Autodesk Fusion 360 part; units mm, degrees
note: some values were not read from the file. Set by a fixed rule: which sketch regions a step uses.
(part 8 of 8)
  spline S993 degree 3 poles (32.1302, -141.7141) (30.6727, -141.6498) (29.2625, -140.8361) (28.4332, -139.581) knots 0 0 0 0 1 1 1 1
  spline S994 degree 3 poles (28.4332, -139.581) (28.0147, -138.9475) (27.7402, -138.2106) (27.6387, -137.4479) knots 0 0 0 0 1 1 1 1
  line L287 (27.6387, -137.4479) -> (27.2253, -124.3326)
  spline S995 degree 3 poles (27.2253, -124.3326) (27.261, -124.1184) (27.1963, -123.8884) (27.0555, -123.7285) knots 0 0 0 0 1 1 1 1
  spline S996 degree 3 poles (27.0555, -123.7285) (26.9778, -123.6402) (26.8783, -123.573) (26.7694, -123.5352) knots 0 0 0 0 1 1 1 1
  spline S997 degree 3 poles (26.7694, -123.5352) (26.6605, -123.4974) (26.5423, -123.489) (26.4295, -123.5111) knots 0 0 0 0 1 1 1 1
  line L288 (26.4295, -123.5111) -> (23.6519, -123.7321)
  spline S998 degree 3 poles (23.6519, -123.7321) (23.5393, -123.6984) (23.4178, -123.6981) (23.3051, -123.7312) knots 0 0 0 0 1 1 1 1
  spline S999 degree 3 poles (23.3051, -123.7312) (23.1924, -123.7643) (23.0888, -123.8306) (23.0094, -123.9206) knots 0 0 0 0 1 1 1 1
  spline S1000 degree 3 poles (23.0094, -123.9206) (22.8811, -124.0659) (22.8198, -124.273) (22.8472, -124.4687) knots 0 0 0 0 1 1 1 1
  line L289 (22.8472, -124.4687) -> (22.8987, -126.766)
  spline S1001 degree 3 poles (36.4911, -133.5813) (36.3024, -133.5736) (36.1111, -133.6504) (35.9788, -133.7913) knots 0 0 0 0 1 1 1 1
  spline S1002 degree 3 poles (35.9788, -133.7913) (35.8464, -133.9322) (35.776, -134.1353) (35.7946, -134.3318) knots 0 0 0 0 1 1 1 1
  spline S1003 degree 3 poles (35.7946, -134.3318) (35.8111, -134.5063) (35.8966, -134.672) (36.0252, -134.7844) knots 0 0 0 0 1 1 1 1
  spline S1004 degree 3 poles (36.0252, -134.7844) (36.1538, -134.8969) (36.3237, -134.9556) (36.4911, -134.9483) knots 0 0 0 0 1 1 1 1
  spline S1005 degree 3 poles (36.4911, -134.9483) (36.6536, -134.9417) (36.8134, -134.8725) (36.9315, -134.7557) knots 0 0 0 0 1 1 1 1
  spline S1006 degree 3 poles (36.9315, -134.7557) (37.0496, -134.6389) (37.1245, -134.4747) (37.1341, -134.305) knots 0 0 0 0 1 1 1 1
  spline S1007 degree 3 poles (37.1341, -134.305) (37.1446, -134.122) (37.0785, -133.9362) (36.9584, -133.8026) knots 0 0 0 0 1 1 1 1
  spline S1008 degree 3 poles (36.9584, -133.8026) (36.8383, -133.669) (36.6663, -133.5888) (36.4911, -133.5813) knots 0 0 0 0 1 1 1 1
  spline S1009 degree 3 poles (46.9493, -133.8297) (46.7703, -133.822) (46.5905, -133.904) (46.4712, -134.0437) knots 0 0 0 0 1 1 1 1
  spline S1010 degree 3 poles (46.4712, -134.0437) (46.3518, -134.1834) (46.294, -134.3772) (46.3113, -134.5636) knots 0 0 0 0 1 1 1 1
  spline S1011 degree 3 poles (46.3113, -134.5636) (46.3267, -134.7281) (46.3999, -134.8866) (46.5162, -134.9984) knots 0 0 0 0 1 1 1 1
  spline S1012 degree 3 poles (46.5162, -134.9984) (46.6326, -135.1102) (46.7914, -135.1734) (46.9493, -135.1665) knots 0 0 0 0 1 1 1 1
  spline S1013 degree 3 poles (46.9493, -135.1665) (47.1029, -135.1599) (47.2524, -135.0871) (47.3591, -134.9713) knots 0 0 0 0 1 1 1 1
  spline S1014 degree 3 poles (47.3591, -134.9713) (47.4657, -134.8554) (47.5292, -134.698) (47.5381, -134.5374) knots 0 0 0 0 1 1 1 1
  spline S1015 degree 3 poles (47.5381, -134.5374) (47.5477, -134.3637) (47.4929, -134.1862) (47.3847, -134.0539) knots 0 0 0 0 1 1 1 1
  spline S1016 degree 3 poles (47.3847, -134.0539) (47.2765, -133.9217) (47.1155, -133.8371) (46.9493, -133.8297) knots 0 0 0 0 1 1 1 1
  spline S1017 degree 3 poles (57.3652, -134.113) (57.1862, -134.1053) (57.0065, -134.1873) (56.8871, -134.327) knots 0 0 0 0 1 1 1 1
  spline S1018 degree 3 poles (56.8871, -134.327) (56.7678, -134.4668) (56.7099, -134.6605) (56.7273, -134.847) knots 0 0 0 0 1 1 1 1
  spline S1019 degree 3 poles (56.7273, -134.847) (56.7426, -135.0114) (56.8159, -135.1699) (56.9322, -135.2817) knots 0 0 0 0 1 1 1 1
  spline S1020 degree 3 poles (56.9322, -135.2817) (57.0485, -135.3935) (57.2073, -135.4567) (57.3652, -135.4498) knots 0 0 0 0 1 1 1 1
  spline S1021 degree 3 poles (57.3652, -135.4498) (57.5189, -135.4432) (57.6683, -135.3705) (57.775, -135.2546) knots 0 0 0 0 1 1 1 1
  spline S1022 degree 3 poles (57.775, -135.2546) (57.8817, -135.1387) (57.9452, -134.9813) (57.954, -134.8208) knots 0 0 0 0 1 1 1 1
  spline S1023 degree 3 poles (57.954, -134.8208) (57.9637, -134.647) (57.9088, -134.4695) (57.8006, -134.3372) knots 0 0 0 0 1 1 1 1
  spline S1024 degree 3 poles (57.8006, -134.3372) (57.6925, -134.205) (57.5315, -134.1204) (57.3652, -134.113) knots 0 0 0 0 1 1 1 1
  spline S1025 degree 3 poles (101.665, -134.9463) (101.4861, -134.9385) (101.3063, -135.0206) (101.187, -135.1603) knots 0 0 0 0 1 1 1 1
  spline S1026 degree 3 poles (101.187, -135.1603) (101.0676, -135.3) (101.0097, -135.4938) (101.0271, -135.6802) knots 0 0 0 0 1 1 1 1
  spline S1027 degree 3 poles (101.0271, -135.6802) (101.0425, -135.8446) (101.1157, -136.0032) (101.232, -136.115) knots 0 0 0 0 1 1 1 1
  spline S1028 degree 3 poles (101.232, -136.115) (101.3483, -136.2268) (101.5072, -136.2899) (101.665, -136.2831) knots 0 0 0 0 1 1 1 1
  spline S1029 degree 3 poles (101.665, -136.2831) (101.8187, -136.2765) (101.9682, -136.2037) (102.0748, -136.0879) knots 0 0 0 0 1 1 1 1
  spline S1030 degree 3 poles (102.0748, -136.0879) (102.1815, -135.972) (102.245, -135.8146) (102.2539, -135.654) knots 0 0 0 0 1 1 1 1
  spline S1031 degree 3 poles (102.2539, -135.654) (102.2635, -135.4803) (102.2086, -135.3027) (102.1005, -135.1705) knots 0 0 0 0 1 1 1 1
  spline S1032 degree 3 poles (102.1005, -135.1705) (101.9923, -135.0382) (101.8313, -134.9537) (101.665, -134.9463) knots 0 0 0 0 1 1 1 1
  spline S1033 degree 3 poles (111.9273, -135.1463) (111.7483, -135.1385) (111.5686, -135.2206) (111.4492, -135.3603) knots 0 0 0 0 1 1 1 1
  spline S1034 degree 3 poles (111.4492, -135.3603) (111.3299, -135.5) (111.272, -135.6938) (111.2894, -135.8802) knots 0 0 0 0 1 1 1 1
  spline S1035 degree 3 poles (111.2894, -135.8802) (111.3047, -136.0446) (111.378, -136.2032) (111.4943, -136.315) knots 0 0 0 0 1 1 1 1
  spline S1036 degree 3 poles (111.4943, -136.315) (111.6106, -136.4268) (111.7695, -136.4899) (111.9273, -136.4831) knots 0 0 0 0 1 1 1 1
  spline S1037 degree 3 poles (111.9273, -136.4831) (112.081, -136.4764) (112.2304, -136.4037) (112.3371, -136.2878) knots 0 0 0 0 1 1 1 1
  spline S1038 degree 3 poles (112.3371, -136.2878) (112.4438, -136.172) (112.5073, -136.0146) (112.5161, -135.854) knots 0 0 0 0 1 1 1 1
  spline S1039 degree 3 poles (112.5161, -135.854) (112.5257, -135.6802) (112.4709, -135.5027) (112.3627, -135.3705) knots 0 0 0 0 1 1 1 1
  spline S1040 degree 3 poles (112.3627, -135.3705) (112.2546, -135.2382) (112.0936, -135.1537) (111.9273, -135.1463) knots 0 0 0 0 1 1 1 1
  spline S1041 degree 2 poles (10.837, -247.6762) (10.81, -245.3593) (10.8501, -244.0773) knots 0 0 0 1 1 1
  spline S1042 degree 3 poles (10.8501, -244.0773) (10.8548, -243.9237) (11.0104, -243.7661) (11.2499, -243.7651) knots 0 0 0 0 1 1 1 1
  spline S1043 degree 3 poles (11.2499, -243.7651) (11.7315, -243.7632) (12.7052, -243.7841) (13.0357, -243.7851) knots 0 0 0 0 1 1 1 1
  spline S1044 degree 3 poles (13.0357, -243.7851) (13.2758, -243.786) (13.4047, -243.6398) (13.4067, -243.5043) knots 0 0 0 0 1 1 1 1
  spline S1045 degree 3 poles (13.4067, -243.5043) (13.4381, -241.3814) (13.4313, -241.3803) (13.4631, -238.9109) knots 0 0 0 0 1 1 1 1
  spline S1046 degree 3 poles (13.4631, -238.9109) (13.4659, -238.6921) (13.2899, -238.5225) (13.0138, -238.5197) knots 0 0 0 0 1 1 1 1
  spline S1047 degree 3 poles (13.0138, -238.5197) (11.7178, -238.5066) (11.93, -238.5149) (11.2628, -238.512) knots 0 0 0 0 1 1 1 1
  spline S1048 degree 3 poles (11.2628, -238.512) (11.1347, -238.5115) (11.0448, -238.4159) (11.0435, -238.2054) knots 0 0 0 0 1 1 1 1
  spline S1049 degree 3 poles (11.0435, -238.2054) (11.0341, -236.7209) (11.0102, -236.7243) (11.0082, -234.862) knots 0 0 0 0 1 1 1 1
  spline S1050 degree 3 poles (11.0082, -234.862) (11.008, -234.6358) (10.9701, -234.5433) (11.2164, -234.546) knots 0 0 0 0 1 1 1 1
  line L290 (11.2164, -234.546) -> (17.2284, -234.6114)
  spline S1051 degree 3 poles (17.2284, -234.6114) (17.5142, -234.6143) (17.5959, -234.6922) (17.5893, -234.9527) knots 0 0 0 0 1 1 1 1
  spline S1052 degree 3 poles (17.5893, -234.9527) (17.5714, -235.6578) (17.819, -236.1257) (18.8656, -236.1706) knots 0 0 0 0 1 1 1 1
  line L291 (18.8656, -236.1706) -> (20.0607, -236.1764)
  spline S1053 degree 2 poles (20.0607, -236.1764) (20.0909, -238.4972) (20.1073, -239.6995) knots 0 0 0 1 1 1
  spline S1054 degree 3 poles (20.1073, -239.6995) (20.109, -239.824) (19.923, -239.9537) (19.7659, -239.9573) knots 0 0 0 0 1 1 1 1
  spline S1055 degree 3 poles (19.7659, -239.9573) (19.0783, -239.9729) (19.0691, -239.9919) (18.4394, -239.9861) knots 0 0 0 0 1 1 1 1
  spline S1056 degree 3 poles (18.4394, -239.9861) (18.2321, -239.9842) (17.9896, -240.1446) (17.9938, -240.3088) knots 0 0 0 0 1 1 1 1
  spline S1057 degree 3 poles (17.9938, -240.3088) (18.0237, -241.5017) (18.0241, -241.5062) (18.0726, -243.1232) knots 0 0 0 0 1 1 1 1
  spline S1058 degree 3 poles (18.0726, -243.1232) (18.0757, -243.2251) (17.962, -243.3631) (17.8333, -243.3632) knots 0 0 0 0 1 1 1 1
  spline S1059 degree 3 poles (17.8333, -243.3632) (17.5642, -243.3634) (17.4937, -243.37) (17.2055, -243.3763) knots 0 0 0 0 1 1 1 1
  spline S1060 degree 3 poles (17.2055, -243.3763) (17.0597, -243.3792) (16.9227, -243.5059) (16.9245, -243.6146) knots 0 0 0 0 1 1 1 1
  line L292 (16.9245, -243.6146) -> (16.9899, -247.6918)
  line L293 (16.9899, -247.6918) -> (10.837, -247.6762)
  spline S1061 degree 2 poles (47.8882, -247.7867) (47.859, -245.8925) (47.8189, -244.6105) knots 0 0 0 1 1 1
  spline S1062 degree 3 poles (47.8189, -244.6105) (47.8142, -244.4569) (47.6586, -244.2992) (47.4191, -244.2983) knots 0 0 0 0 1 1 1 1
  spline S1063 degree 3 poles (47.4191, -244.2983) (46.9375, -244.2963) (45.9638, -244.3173) (45.6333, -244.3182) knots 0 0 0 0 1 1 1 1
  spline S1064 degree 3 poles (45.6333, -244.3182) (45.3932, -244.3192) (45.2643, -244.173) (45.2623, -244.0375) knots 0 0 0 0 1 1 1 1
  spline S1065 degree 3 poles (45.2623, -244.0375) (45.2309, -241.9146) (45.2377, -241.9135) (45.2059, -239.444) knots 0 0 0 0 1 1 1 1
  spline S1066 degree 3 poles (45.2059, -239.444) (45.2031, -239.2253) (45.3791, -239.0557) (45.6552, -239.0529) knots 0 0 0 0 1 1 1 1
  spline S1067 degree 3 poles (45.6552, -239.0529) (46.9512, -239.0398) (46.739, -239.0481) (47.4062, -239.0452) knots 0 0 0 0 1 1 1 1
  spline S1068 degree 3 poles (47.4062, -239.0452) (47.5343, -239.0447) (47.6242, -238.9491) (47.6255, -238.7386) knots 0 0 0 0 1 1 1 1
  spline S1069 degree 3 poles (47.6255, -238.7386) (47.6349, -237.254) (47.6588, -237.2575) (47.6608, -235.3952) knots 0 0 0 0 1 1 1 1
  spline S1070 degree 3 poles (47.6608, -235.3952) (47.661, -235.1689) (47.6989, -235.0765) (47.4526, -235.0791) knots 0 0 0 0 1 1 1 1
  line L294 (47.4526, -235.0791) -> (41.4406, -235.1446)
  spline S1071 degree 3 poles (41.4406, -235.1446) (41.1548, -235.1475) (41.1393, -235.1728) (41.1459, -235.4334) knots 0 0 0 0 1 1 1 1
  spline S1072 degree 3 poles (41.1459, -235.4334) (41.1638, -236.1385) (40.9162, -236.5277) (39.8696, -236.5726) knots 0 0 0 0 1 1 1 1
  line L295 (39.8696, -236.5726) -> (38.5255, -236.5259)
  spline S1073 degree 2 poles (38.5255, -236.5259) (38.5118, -238.5714) (38.4955, -239.7736) knots 0 0 0 1 1 1
  spline S1074 degree 3 poles (38.4955, -239.7736) (38.4938, -239.8982) (38.6797, -240.0279) (38.8369, -240.0315) knots 0 0 0 0 1 1 1 1
  spline S1075 degree 3 poles (38.8369, -240.0315) (39.5245, -240.0471) (39.0039, -240.053) (39.6336, -240.0472) knots 0 0 0 0 1 1 1 1
  spline S1076 degree 3 poles (39.6336, -240.0472) (39.8409, -240.0452) (40.0781, -240.2056) (40.0793, -240.3698) knots 0 0 0 0 1 1 1 1
  spline S1077 degree 3 poles (40.0793, -240.3698) (40.0997, -243.2891) (40.0793, -240.3698) (40.0997, -243.2891) knots 0 0 0 0 1 1 1 1
  spline S1078 degree 3 poles (40.0997, -243.2891) (40.1004, -243.3911) (40.2104, -243.5291) (40.3391, -243.5292) knots 0 0 0 0 1 1 1 1
  spline S1079 degree 3 poles (40.3391, -243.5292) (40.6082, -243.5294) (40.6787, -243.5359) (40.9668, -243.5422) knots 0 0 0 0 1 1 1 1
  spline S1080 degree 3 poles (40.9668, -243.5422) (41.1127, -243.5451) (41.2482, -243.6718) (41.2479, -243.7806) knots 0 0 0 0 1 1 1 1
  line L296 (41.2479, -243.7806) -> (41.2883, -247.7892)
  line L297 (41.2883, -247.7892) -> (47.8882, -247.7867)
  spline S1081 degree 3 poles (7.9694, -248.7095) (6.13, -246.5222) (6.2347, -236.0812) (8.0811, -233.6481) knots 0 0 0 0 1 1 1 1
  spline S1082 degree 3 poles (8.0811, -233.6481) (10.5104, -230.4468) (17.2788, -229.16) (22.0462, -228.4083) knots 0 0 0 0 1 1 1 1
  spline S1083 degree 3 poles (22.0462, -228.4083) (24.6723, -227.9942) (34.366, -228.0312) (36.3491, -228.4083) knots 0 0 0 0 1 1 1 1
  spline S1084 degree 3 poles (36.3491, -228.4083) (41.2162, -229.3338) (47.3408, -230.9515) (49.7581, -232.9453) knots 0 0 0 0 1 1 1 1
  spline S1085 degree 3 poles (49.7581, -232.9453) (52.8167, -235.4681) (52.4282, -246.7854) (50.3256, -249.234) knots 0 0 0 0 1 1 1 1
  spline S1086 degree 3 poles (50.3256, -249.234) (47.576, -252.4361) (40.6483, -252.9931) (35.4495, -254.2169) knots 0 0 0 0 1 1 1 1
  spline S1087 degree 3 poles (35.4495, -254.2169) (33.2181, -254.7421) (24.4667, -254.5045) (22.8569, -254.2015) knots 0 0 0 0 1 1 1 1
  spline S1088 degree 3 poles (22.8569, -254.2015) (17.5924, -253.2105) (10.1045, -251.2484) (7.9694, -248.7095) knots 0 0 0 0 1 1 1 1
  spline S1089 degree 3 poles (29.1976, -234.073) (31.1453, -234.0759) (32.8241, -235.8872) (32.8396, -237.6921) knots 0 0 0 0 1 1 1 1
  spline S1090 degree 3 poles (32.8396, -237.6921) (32.8528, -239.2378) (31.2151, -241.3793) (29.2639, -241.3637) knots 0 0 0 0 1 1 1 1
  spline S1091 degree 3 poles (29.2639, -241.3637) (27.2598, -241.3477) (25.6544, -239.1221) (25.6881, -237.5348) knots 0 0 0 0 1 1 1 1
  spline S1092 degree 3 poles (25.6881, -237.5348) (25.7252, -235.7929) (27.3293, -234.0703) (29.1976, -234.073) knots 0 0 0 0 1 1 1 1
  spline S1093 degree 3 poles (29.1645, -230.3227) (28.7036, -230.3295) (28.2258, -230.7707) (28.2375, -231.1357) knots 0 0 0 0 1 1 1 1
  spline S1094 degree 3 poles (28.2375, -231.1357) (28.2502, -231.5312) (28.7982, -231.9953) (29.297, -231.9749) knots 0 0 0 0 1 1 1 1
  spline S1095 degree 3 poles (29.297, -231.9749) (29.7514, -231.9564) (30.1775, -231.4958) (30.1578, -231.1357) knots 0 0 0 0 1 1 1 1
  spline S1096 degree 3 poles (30.1578, -231.1357) (30.1372, -230.759) (29.6406, -230.3162) (29.1645, -230.3227) knots 0 0 0 0 1 1 1 1
  spline S1097 degree 3 poles (29.0652, -243.4355) (28.6043, -243.4423) (28.1265, -243.8835) (28.1382, -244.2485) knots 0 0 0 0 1 1 1 1
  spline S1098 degree 3 poles (28.1382, -244.2485) (28.1509, -244.644) (28.6989, -245.1081) (29.1977, -245.0877) knots 0 0 0 0 1 1 1 1
  spline S1099 degree 3 poles (29.1977, -245.0877) (29.6521, -245.0692) (30.0782, -244.6086) (30.0585, -244.2485) knots 0 0 0 0 1 1 1 1
  spline S1100 degree 3 poles (30.0585, -244.2485) (30.0378, -243.8718) (29.5412, -243.429) (29.0652, -243.4355) knots 0 0 0 0 1 1 1 1
  spline S1101 degree 3 poles (22.5759, -236.748) (22.115, -236.7548) (21.6372, -237.1959) (21.6489, -237.561) knots 0 0 0 0 1 1 1 1
  spline S1102 degree 3 poles (21.6489, -237.561) (21.6616, -237.9565) (22.2096, -238.4206) (22.7084, -238.4002) knots 0 0 0 0 1 1 1 1
  spline S1103 degree 3 poles (22.7084, -238.4002) (23.1628, -238.3817) (23.5889, -237.9211) (23.5692, -237.561) knots 0 0 0 0 1 1 1 1
  spline S1104 degree 3 poles (23.5692, -237.561) (23.5486, -237.1842) (23.052, -236.7415) (22.5759, -236.748) knots 0 0 0 0 1 1 1 1
  spline S1105 degree 3 poles (35.5545, -236.8267) (35.0935, -236.8334) (34.6157, -237.2746) (34.6275, -237.6397) knots 0 0 0 0 1 1 1 1
  spline S1106 degree 3 poles (34.6275, -237.6397) (34.6401, -238.0352) (35.1881, -238.4993) (35.6869, -238.4789) knots 0 0 0 0 1 1 1 1
  spline S1107 degree 3 poles (35.6869, -238.4789) (36.1414, -238.4604) (36.5675, -237.9998) (36.5477, -237.6397) knots 0 0 0 0 1 1 1 1
  spline S1108 degree 3 poles (36.5477, -237.6397) (36.5271, -237.2629) (36.0305, -236.8202) (35.5545, -236.8267) knots 0 0 0 0 1 1 1 1
  spline S1109 degree 3 poles (18.785, -250.3459) (18.748, -249.1063) (18.7991, -248.5212) (18.7685, -247.3694) knots 0 0 0 0 1 1 1 1
  spline S1110 degree 3 poles (18.7685, -247.3694) (18.7615, -247.1095) (18.9371, -246.8518) (19.381, -246.858) knots 0 0 0 0 1 1 1 1
  spline S1111 degree 3 poles (19.381, -246.858) (25.3461, -246.9402) (29.4591, -246.8339) (38.9481, -246.8579) knots 0 0 0 0 1 1 1 1
  spline S1112 degree 3 poles (38.9481, -246.8579) (39.4808, -246.8589) (39.8824, -246.9253) (39.8917, -247.2382) knots 0 0 0 0 1 1 1 1
  spline S1113 degree 3 poles (39.8917, -247.2382) (39.9326, -248.6175) (39.9249, -249.0855) (39.9579, -250.8311) knots 0 0 0 0 1 1 1 1
  spline S1114 degree 3 poles (39.9579, -250.8311) (39.9639, -251.1444) (39.3598, -251.1674) (38.8847, -251.1733) knots 0 0 0 0 1 1 1 1
  spline S1115 degree 3 poles (38.8847, -251.1733) (31.2086, -251.2686) (22.9608, -251.1294) (19.6127, -251.1458) knots 0 0 0 0 1 1 1 1
  spline S1116 degree 3 poles (19.6127, -251.1458) (18.9796, -251.1794) (18.7993, -250.8065) (18.785, -250.3459) knots 0 0 0 0 1 1 1 1
  spline S1117 degree 3 poles (106.8581, -62.4361) (107.4615, -63.4086) (126.8754, -59.2722) (130.1181, -59.5077) knots 0 0 0 0 1 1 1 1
  spline S1118 degree 3 poles (130.1181, -59.5077) (134.3606, -59.8157) (139.0785, -60.7934) (144.166, -60.6989) knots 0 0 0 0 1 1 1 1
  spline S1119 degree 3 poles (144.166, -60.6989) (145.4225, -60.6737) (146.6093, -58.2172) (146.1712, -58.2172) knots 0 0 0 0 1 1 1 1
  line L298 (146.1712, -58.2172) -> (144.4491, -58.1794)
  line L299 (144.4491, -58.1794) -> (144.5317, -54.8538)
  line L300 (144.5317, -54.8538) -> (148.9077, -54.8665)
  spline S1120 degree 3 poles (148.9077, -54.8665) (150.9289, -54.8707) (153.9314, -45.6994) (153.2011, -43.1776) knots 0 0 0 0 1 1 1 1
  spline S1121 degree 2 poles (153.2011, -43.1776) (152.9643, -42.3602) (131.8833, -41.4876) knots 0 0 0 1 1 1
  line L301 (131.8833, -41.4876) -> (132.3596, -27.2637)
  spline S1122 degree 2 poles (132.3596, -27.2637) (152.4979, -28.1981) (153.5195, -27.5927) knots 0 0 0 1 1 1
  spline S1123 degree 3 poles (153.5195, -27.5927) (155.6549, -26.3272) (151.6676, -14.9886) (150.4764, -14.9732) knots 0 0 0 0 1 1 1 1
  line L302 (150.4764, -14.9732) -> (146.6548, -14.9236)
  line L303 (146.6548, -14.9236) -> (146.6428, -11.4244)
  line L304 (146.6428, -11.4244) -> (147.9756, -11.4117)
  spline S1124 degree 2 poles (147.9756, -11.4117) (149.5302, -11.3991) (145.4515, -8.5825) knots 0 0 0 1 1 1
  spline S1125 degree 2 poles (145.4515, -8.5825) (137.5261, -9.626) (133.562, -9.3767) knots 0 0 0 1 1 1
  spline S1126 degree 3 poles (133.562, -9.3767) (125.1006, -8.8445) (109.1577, -3.6312) (108.5564, -4.5126) knots 0 0 0 0 1 1 1 1
  spline S1127 degree 3 poles (108.5564, -4.5126) (107.7409, -5.708) (114.1986, -16.9111) (115.5391, -23.5721) knots 0 0 0 0 1 1 1 1
  spline S1128 degree 2 poles (115.5391, -23.5721) (116.1079, -26.3984) (115.9459, -32.2282) knots 0 0 0 1 1 1
  line L305 (115.9459, -32.2282) -> (117.8444, -32.2313)
  line L306 (117.8444, -32.2313) -> (117.8981, -35.9809)
  line L307 (117.8981, -35.9809) -> (116.0412, -36.0359)
  spline S1129 degree 2 poles (116.0412, -36.0359) (116.1197, -41.6582) (115.256, -44.2203) knots 0 0 0 1 1 1
  spline S1130 degree 3 poles (115.256, -44.2203) (113.7246, -48.7631) (106.2438, -61.4466) (106.8581, -62.4361) knots 0 0 0 0 1 1 1 1
  spline S1131 degree 3 poles (118.1745, -48.0159) (119.0012, -48.0327) (125.7923, -54.9365) (125.5975, -56.246) knots 0 0 0 0 1 1 1 1
  spline S1132 degree 3 poles (125.5975, -56.246) (125.4017, -57.5625) (113.7841, -58.9903) (113.0869, -57.9833) knots 0 0 0 0 1 1 1 1
  spline S1133 degree 3 poles (113.0869, -57.9833) (112.4893, -57.1201) (117.1764, -47.9978) (118.1745, -48.0159) knots 0 0 0 0 1 1 1 1
  spline S1134 degree 3 poles (115.2217, -9.406) (114.805, -10.0096) (118.3286, -19.4875) (119.2901, -19.5024) knots 0 0 0 0 1 1 1 1
  spline S1135 degree 3 poles (119.2901, -19.5024) (120.1689, -19.515) (127.7392, -13.1963) (127.3344, -11.8338) knots 0 0 0 0 1 1 1 1
  spline S1136 degree 3 poles (127.3344, -11.8338) (127.0183, -10.7697) (115.6902, -8.7274) (115.2217, -9.406) knots 0 0 0 0 1 1 1 1
  spline S1137 degree 3 poles (23.635, -150.8434) (24.5086, -148.6901) (26.1171, -146.8428) (28.1299, -145.6814) knots 0 0 0 0 1 1 1 1
  spline S1138 degree 3 poles (28.1299, -145.6814) (30.1426, -144.5201) (32.5469, -144.0519) (34.8484, -144.3733) knots 0 0 0 0 1 1 1 1
  spline S1139 degree 3 poles (34.8484, -144.3733) (52.6997, -145.8548) (70.5006, -147.9437) (88.21, -150.6351) knots 0 0 0 0 1 1 1 1
  spline S1140 degree 3 poles (88.21, -150.6351) (96.7525, -151.9334) (105.2738, -153.3718) (113.7692, -154.9496) knots 0 0 0 0 1 1 1 1
  line L308 (113.7692, -154.9496) -> (119.5937, -159.5032)
  spline S1141 degree 3 poles (119.5937, -159.5032) (120.3382, -160.7189) (120.741, -162.1415) (120.7442, -163.5672) knots 0 0 0 0 1 1 1 1
  spline S1142 degree 3 poles (120.7442, -163.5672) (120.7472, -164.9195) (120.3916, -166.2711) (119.7232, -167.4468) knots 0 0 0 0 1 1 1 1
  line L309 (119.7232, -167.4468) -> (112.4351, -171.7089)
  spline S1143 degree 3 poles (112.4351, -171.7089) (103.5371, -171.4668) (94.6435, -171.0669) (85.7597, -170.5096) knots 0 0 0 0 1 1 1 1
  spline S1144 degree 3 poles (85.7597, -170.5096) (67.4605, -169.3616) (49.2034, -167.5449) (31.0368, -165.0646) knots 0 0 0 0 1 1 1 1
  spline S1145 degree 3 poles (31.0368, -165.0646) (28.0767, -164.3852) (25.4542, -162.3573) (24.052, -159.6632) knots 0 0 0 0 1 1 1 1
  spline S1146 degree 3 poles (24.052, -159.6632) (22.6499, -156.9692) (22.4933, -153.6578) (23.635, -150.8434) knots 0 0 0 0 1 1 1 1
  spline S1147 degree 3 poles (26.953, -153.0854) (26.6067, -153.0691) (26.2584, -153.2223) (26.0288, -153.4822) knots 0 0 0 0 1 1 1 1
  spline S1148 degree 3 poles (26.0288, -153.4822) (25.7992, -153.7422) (25.6904, -154.102) (25.7279, -154.4467) knots 0 0 0 0 1 1 1 1
  spline S1149 degree 3 poles (25.7279, -154.4467) (25.7605, -154.7462) (25.9022, -155.0338) (26.1254, -155.236) knots 0 0 0 0 1 1 1 1
  spline S1150 degree 3 poles (26.1254, -155.236) (26.3486, -155.4381) (26.6523, -155.5509) (26.953, -155.5358) knots 0 0 0 0 1 1 1 1
  spline S1151 degree 3 poles (26.953, -155.5358) (27.2117, -155.5236) (27.4635, -155.4156) (27.657, -155.2433) knots 0 0 0 0 1 1 1 1
  spline S1152 degree 3 poles (27.657, -155.2433) (27.8504, -155.0709) (27.9852, -154.8355) (28.042, -154.5828) knots 0 0 0 0 1 1 1 1
  spline S1153 degree 3 poles (28.042, -154.5828) (28.1192, -154.2398) (28.049, -153.8643) (27.8451, -153.578) knots 0 0 0 0 1 1 1 1
  spline S1154 degree 3 poles (27.8451, -153.578) (27.6411, -153.2916) (27.3042, -153.1017) (26.953, -153.0854) knots 0 0 0 0 1 1 1 1
  spline S1155 degree 3 poles (48.9034, -160.1299) (48.8627, -160.2823) (48.8293, -160.4376) (48.8273, -160.5953) knots 0 0 0 0 1 1 1 1
  spline S1156 degree 3 poles (48.8273, -160.5953) (48.8253, -160.753) (48.8562, -160.9135) (48.9377, -161.0488) knots 0 0 0 0 1 1 1 1
  spline S1157 degree 3 poles (48.9377, -161.0488) (49.0524, -161.2395) (49.2679, -161.3654) (49.4903, -161.3719) knots 0 0 0 0 1 1 1 1
  spline S1158 degree 3 poles (49.4903, -161.3719) (49.7127, -161.38) (49.9351, -161.2651) (50.0607, -161.0814) knots 0 0 0 0 1 1 1 1
  spline S1159 degree 3 poles (50.0607, -161.0814) (51.4229, -159.8943) (52.2579, -158.123) (52.3068, -156.3169) knots 0 0 0 0 1 1 1 1
  spline S1160 degree 3 poles (52.3068, -156.3169) (52.3439, -154.9506) (51.9504, -153.5989) (51.3539, -152.3692) knots 0 0 0 0 1 1 1 1
  spline S1161 degree 3 poles (51.3539, -152.3692) (51.2759, -152.2082) (51.1934, -152.0477) (51.0788, -151.9107) knots 0 0 0 0 1 1 1 1
  spline S1162 degree 3 poles (51.0788, -151.9107) (50.9641, -151.7738) (50.8134, -151.6606) (50.6393, -151.6206) knots 0 0 0 0 1 1 1 1
  spline S1163 degree 3 poles (50.6393, -151.6206) (50.5334, -151.5962) (50.4213, -151.6003) (50.3173, -151.6329) knots 0 0 0 0 1 1 1 1
  spline S1164 degree 3 poles (50.3173, -151.6329) (50.2133, -151.6655) (50.1177, -151.7225) (50.0426, -151.8012) knots 0 0 0 0 1 1 1 1
  spline S1165 degree 3 poles (50.0426, -151.8012) (49.9676, -151.8798) (49.9133, -151.978) (49.8868, -152.0832) knots 0 0 0 0 1 1 1 1
  spline S1166 degree 3 poles (49.8868, -152.0832) (49.8603, -152.1883) (49.8615, -152.3008) (49.8906, -152.405) knots 0 0 0 0 1 1 1 1
  spline S1167 degree 3 poles (49.8906, -152.405) (50.1218, -153.7984) (50.1335, -155.228) (49.9248, -156.625) knots 0 0 0 0 1 1 1 1
  spline S1168 degree 3 poles (49.9248, -156.625) (49.7444, -157.8322) (49.4, -159.015) (48.9038, -160.1302) knots 0 0 0 0 1 1 1 1
  spline S1169 degree 3 poles (48.9038, -160.1302) (48.9037, -160.1307) (48.9036, -160.1312) (48.9035, -160.1317) knots 0 0 0 0 1 1 1 1
  line L310 (48.9035, -160.1317) -> (48.9034, -160.1299)
  spline S1170 degree 3 poles (61.3829, -161.6031) (61.3422, -161.7554) (61.3088, -161.9107) (61.3068, -162.0684) knots 0 0 0 0 1 1 1 1
  spline S1171 degree 3 poles (61.3068, -162.0684) (61.3047, -162.2261) (61.3357, -162.3866) (61.4171, -162.5219) knots 0 0 0 0 1 1 1 1
  spline S1172 degree 3 poles (61.4171, -162.5219) (61.5319, -162.7126) (61.7473, -162.8385) (61.9698, -162.845) knots 0 0 0 0 1 1 1 1
  spline S1173 degree 3 poles (61.9698, -162.845) (62.1922, -162.8532) (62.4146, -162.7383) (62.5402, -162.5545) knots 0 0 0 0 1 1 1 1
  spline S1174 degree 3 poles (62.5402, -162.5545) (63.9023, -161.3674) (64.7374, -159.5962) (64.7863, -157.79) knots 0 0 0 0 1 1 1 1
  spline S1175 degree 3 poles (64.7863, -157.79) (64.8233, -156.4237) (64.4299, -155.0721) (63.8334, -153.8423) knots 0 0 0 0 1 1 1 1
  spline S1176 degree 3 poles (63.8334, -153.8423) (63.7554, -153.6814) (63.6729, -153.5208) (63.5582, -153.3839) knots 0 0 0 0 1 1 1 1
  spline S1177 degree 3 poles (63.5582, -153.3839) (63.4436, -153.247) (63.2929, -153.1337) (63.1187, -153.0938) knots 0 0 0 0 1 1 1 1
  spline S1178 degree 3 poles (63.1187, -153.0938) (63.0129, -153.0693) (62.9008, -153.0734) (62.7968, -153.106) knots 0 0 0 0 1 1 1 1
  spline S1179 degree 3 poles (62.7968, -153.106) (62.6928, -153.1386) (62.5971, -153.1957) (62.5221, -153.2743) knots 0 0 0 0 1 1 1 1
  spline S1180 degree 3 poles (62.5221, -153.2743) (62.447, -153.353) (62.3928, -153.4512) (62.3663, -153.5563) knots 0 0 0 0 1 1 1 1
  spline S1181 degree 3 poles (62.3663, -153.5563) (62.3398, -153.6614) (62.341, -153.7739) (62.37, -153.8782) knots 0 0 0 0 1 1 1 1
  spline S1182 degree 3 poles (62.37, -153.8782) (62.6013, -155.2715) (62.6129, -156.7011) (62.4043, -158.0981) knots 0 0 0 0 1 1 1 1
  spline S1183 degree 3 poles (62.4043, -158.0981) (62.2239, -159.3054) (61.8795, -160.4881) (61.3833, -161.6034) knots 0 0 0 0 1 1 1 1
  spline S1184 degree 3 poles (61.3833, -161.6034) (61.3832, -161.6039) (61.383, -161.6044) (61.3829, -161.6049) knots 0 0 0 0 1 1 1 1
  line L311 (61.3829, -161.6049) -> (61.3829, -161.6031)
  spline S1185 degree 3 poles (73.8962, -162.8544) (73.8554, -163.0067) (73.822, -163.162) (73.82, -163.3197) knots 0 0 0 0 1 1 1 1
  spline S1186 degree 3 poles (73.82, -163.3197) (73.818, -163.4774) (73.849, -163.6384) (73.9304, -163.7732) knots 0 0 0 0 1 1 1 1
  spline S1187 degree 3 poles (73.9304, -163.7732) (74.0452, -163.9639) (74.2606, -164.0898) (74.483, -164.0963) knots 0 0 0 0 1 1 1 1
  spline S1188 degree 3 poles (74.483, -164.0963) (74.7055, -164.1045) (74.9278, -163.9896) (75.0535, -163.8058) knots 0 0 0 0 1 1 1 1
  spline S1189 degree 3 poles (75.0535, -163.8058) (76.4156, -162.6187) (77.2506, -160.8475) (77.2995, -159.0413) knots 0 0 0 0 1 1 1 1
  spline S1190 degree 3 poles (77.2995, -159.0413) (77.3366, -157.675) (76.9432, -156.3234) (76.3467, -155.0936) knots 0 0 0 0 1 1 1 1
  spline S1191 degree 3 poles (76.3467, -155.0936) (76.2687, -154.9327) (76.1862, -154.7721) (76.0715, -154.6352) knots 0 0 0 0 1 1 1 1
  spline S1192 degree 3 poles (76.0715, -154.6352) (75.9568, -154.4983) (75.8062, -154.385) (75.632, -154.3451) knots 0 0 0 0 1 1 1 1
  spline S1193 degree 3 poles (75.632, -154.3451) (75.5262, -154.3206) (75.414, -154.3247) (75.3101, -154.3573) knots 0 0 0 0 1 1 1 1
  spline S1194 degree 3 poles (75.3101, -154.3573) (75.206, -154.3899) (75.1104, -154.447) (75.0354, -154.5256) knots 0 0 0 0 1 1 1 1
  spline S1195 degree 3 poles (75.0354, -154.5256) (74.9603, -154.6043) (74.9061, -154.7024) (74.8795, -154.8076) knots 0 0 0 0 1 1 1 1
  spline S1196 degree 3 poles (74.8795, -154.8076) (74.8531, -154.9127) (74.8543, -155.0252) (74.8833, -155.1295) knots 0 0 0 0 1 1 1 1
  spline S1197 degree 3 poles (74.8833, -155.1295) (75.1146, -156.5228) (75.1262, -157.9524) (74.9175, -159.3494) knots 0 0 0 0 1 1 1 1
  spline S1198 degree 3 poles (74.9175, -159.3494) (74.7372, -160.5567) (74.3927, -161.7394) (73.8966, -162.8547) knots 0 0 0 0 1 1 1 1
  spline S1199 degree 3 poles (73.8966, -162.8547) (73.8965, -162.8552) (73.8963, -162.8557) (73.8962, -162.8562) knots 0 0 0 0 1 1 1 1
  line L312 (73.8962, -162.8562) -> (73.8962, -162.8544)
  spline S1200 degree 3 poles (86.3132, -163.9132) (86.2725, -164.0656) (86.239, -164.2209) (86.2371, -164.3786) knots 0 0 0 0 1 1 1 1
  spline S1201 degree 3 poles (86.2371, -164.3786) (86.235, -164.5363) (86.266, -164.6968) (86.3474, -164.8321) knots 0 0 0 0 1 1 1 1
  spline S1202 degree 3 poles (86.3474, -164.8321) (86.4622, -165.0228) (86.6776, -165.1487) (86.9001, -165.1552) knots 0 0 0 0 1 1 1 1
  spline S1203 degree 3 poles (86.9001, -165.1552) (87.1225, -165.1633) (87.3449, -165.0484) (87.4705, -164.8647) knots 0 0 0 0 1 1 1 1
  spline S1204 degree 3 poles (87.4705, -164.8647) (88.8326, -163.6776) (89.6676, -161.9063) (89.7166, -160.1002) knots 0 0 0 0 1 1 1 1
  spline S1205 degree 3 poles (89.7166, -160.1002) (89.7536, -158.7339) (89.3602, -157.3822) (88.7637, -156.1525) knots 0 0 0 0 1 1 1 1
  spline S1206 degree 3 poles (88.7637, -156.1525) (88.6857, -155.9915) (88.6032, -155.831) (88.4885, -155.694) knots 0 0 0 0 1 1 1 1
  spline S1207 degree 3 poles (88.4885, -155.694) (88.3739, -155.5571) (88.2232, -155.4439) (88.049, -155.4039) knots 0 0 0 0 1 1 1 1
  spline S1208 degree 3 poles (88.049, -155.4039) (87.9432, -155.3795) (87.8311, -155.3836) (87.7271, -155.4162) knots 0 0 0 0 1 1 1 1
  spline S1209 degree 3 poles (87.7271, -155.4162) (87.623, -155.4488) (87.5274, -155.5059) (87.4524, -155.5845) knots 0 0 0 0 1 1 1 1
  spline S1210 degree 3 poles (87.4524, -155.5845) (87.3773, -155.6631) (87.3231, -155.7613) (87.2966, -155.8665) knots 0 0 0 0 1 1 1 1
  spline S1211 degree 3 poles (87.2966, -155.8665) (87.2701, -155.9716) (87.2713, -156.0841) (87.3003, -156.1888) knots 0 0 0 0 1 1 1 1
  spline S1212 degree 3 poles (87.3003, -156.1888) (87.5316, -157.5821) (87.5432, -159.0117) (87.3345, -160.4087) knots 0 0 0 0 1 1 1 1
  spline S1213 degree 3 poles (87.3345, -160.4087) (87.1542, -161.616) (86.8098, -162.7987) (86.3136, -163.914) knots 0 0 0 0 1 1 1 1
  spline S1214 degree 3 poles (86.3136, -163.914) (86.3135, -163.9145) (86.3133, -163.915) (86.3132, -163.9155) knots 0 0 0 0 1 1 1 1
  line L313 (86.3132, -163.9155) -> (86.3132, -163.9132)
  line L314 (112.5713, -165.2288) -> (107.1329, -166.071)
  spline S1215 degree 3 poles (107.1329, -166.071) (106.0422, -166.113) (104.9428, -165.6379) (104.2257, -164.815) knots 0 0 0 0 1 1 1 1
  spline S1216 degree 3 poles (104.2257, -164.815) (103.5086, -163.9922) (103.1884, -162.8382) (103.3789, -161.7635) knots 0 0 0 0 1 1 1 1
  spline S1217 degree 3 poles (103.3789, -161.7635) (103.5446, -160.8286) (104.0893, -159.9667) (104.8625, -159.4157) knots 0 0 0 0 1 1 1 1
  spline S1218 degree 3 poles (104.8625, -159.4157) (105.6357, -158.8647) (106.6282, -158.6311) (107.566, -158.7796) knots 0 0 0 0 1 1 1 1
  line L315 (107.566, -158.7796) -> (112.7879, -160.416)
  line L316 (112.7879, -160.416) -> (112.5713, -165.2288)
  spline S1219 degree 3 poles (116.566, -162.4374) (116.1771, -162.4353) (115.7784, -162.4292) (115.412, -162.5583) knots 0 0 0 0 1 1 1 1
  spline S1220 degree 3 poles (115.412, -162.5583) (115.2288, -162.6236) (115.056, -162.7234) (114.9206, -162.8627) knots 0 0 0 0 1 1 1 1
  spline S1221 degree 3 poles (114.9206, -162.8627) (114.7851, -163.0021) (114.6886, -163.1826) (114.6649, -163.3757) knots 0 0 0 0 1 1 1 1
  spline S1222 degree 3 poles (114.6649, -163.3757) (114.6372, -163.6014) (114.7113, -163.8335) (114.8471, -164.0157) knots 0 0 0 0 1 1 1 1
  spline S1223 degree 3 poles (114.8471, -164.0157) (114.9829, -164.1978) (115.177, -164.3323) (115.3878, -164.417) knots 0 0 0 0 1 1 1 1
  spline S1224 degree 3 poles (115.3878, -164.417) (115.8096, -164.5865) (116.281, -164.5629) (116.7344, -164.5307) knots 0 0 0 0 1 1 1 1
  spline S1225 degree 3 poles (116.7344, -164.5307) (117.1035, -164.5062) (117.4827, -164.4724) (117.8145, -164.3086) knots 0 0 0 0 1 1 1 1
  spline S1226 degree 3 poles (117.8145, -164.3086) (117.9804, -164.2267) (118.1319, -164.1118) (118.2426, -163.9635) knots 0 0 0 0 1 1 1 1
  spline S1227 degree 3 poles (118.2426, -163.9635) (118.3533, -163.8151) (118.4215, -163.6326) (118.4189, -163.4476) knots 0 0 0 0 1 1 1 1
  spline S1228 degree 3 poles (118.4189, -163.4476) (118.4162, -163.2516) (118.3339, -163.0605) (118.2067, -162.9112) knots 0 0 0 0 1 1 1 1
  spline S1229 degree 3 poles (118.2067, -162.9112) (118.0794, -162.7617) (117.9095, -162.6525) (117.727, -162.5804) knots 0 0 0 0 1 1 1 1
  spline S1230 degree 3 poles (117.727, -162.5804) (117.362, -162.4361) (116.9583, -162.439) (116.566, -162.4369) knots 0 0 0 0 1 1 1 1
  line L317 (116.566, -162.4369) -> (116.566, -162.4374)
extrude "Extrude2" add sketch "Sketch2" along normal blind 3.5 separate body contours S1137 S1138 S1139 S1140 L308 S1141 S1142 L309 S1143 S1144 S1145 S1146 makes body 19
